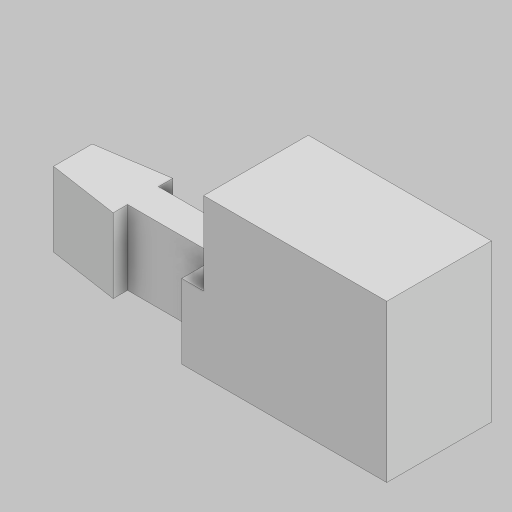
# Autodesk Inventor part: Tenon2
Saved by Autodesk Inventor 2023 (Build 270158000, 158)
## iProperties
Created: 2026-02-15
Part Number: Tenon2
Material: Genérico
Document SubType Name: Modeling
Designer: MARTIN MAESTRE
Density: 1 g/cm^3
Appearance: Valor por defecto
Author: MARTIN MAESTRE
Autodesk Inventor part; units mm, degrees
ref_plane "YZ Plane" through (0, 0, 0) normal (1, 0, 0) x (0, 1, 0)
ref_plane "XZ Plane" through (0, 0, 0) normal (0, 1, 0) x (-1, 0, 0)
ref_plane "XY Plane" through (0, 0, 0) normal (0, 0, 1) x (1, 0, 0)
sketch "Boceto1" plane through (0, 0, 0) normal (0, 0, 1) x (1, 0, 0)
  line L0 (0, 0) -> (140, 0)
  line L1 (140, 0) -> (140, 60)
  line L2 (140, 60) -> (0, 60)
  line L3 (0, 60) -> (0, 0)
  dimension "d0" = 140
  dimension "d1" = 60
  constraints: 8 end point, 3 perpendicular, 1 horizontal
  measures "d0" distance of L0.start L0.end
  measures "d1" distance of L0.end L1.end
extrude "Extrusión1" add sketch "Boceto1" along normal blind 40
sketch "Boceto2" plane through (0, 60, 0) normal (0, 1, 0) x (1, 0, 0)
  line L0 (140, -40) -> (0, -40) projected
  line L1 (0, 0) -> (0, -40)
  line L2 (140, 0) -> (0, 0) projected
  line L3 (0, 0) -> (70, 0)
  line L4 (0, 0) -> (70, 0) construction
  line L5 (70, 0) -> (70, -40)
  line L6 (0, -40) -> (70, -40)
  dimension "d4" = 70
  dimension "d5" = 0
  constraints: 10 end point, 3 collinear, 1 horizontal, 1 midpoint, 1 vertical
  measures "d4" distance of L1.start L3.end
  measures "d5" distance between parallel lines of L3 L4
extrude "Extrusión2" cut sketch "Boceto2" against normal blind 31.6
sketch "Boceto3" plane through (0, 0, 0) normal (0, -1, 0) x (1, 0, 0)
  line L0 (0, 0) -> (140, 0) projected
  line L1 (0, 0) -> (0, 12.6)
  line L2 (0, 0) -> (0, 40) projected
  line L3 (0, 12.6) -> (0, 27.4) construction
  line L4 (0, 27.4) -> (0, 40)
  line L5 (0, 0) -> (26.8, 0)
  line L6 (26.8, 0) -> (26.8, 8.6) construction
  line L7 (0, 12.6) -> (26.8, 8.6)
  line L8 (26.8, 0) -> (26.8, 8.6)
  line L9 (26.8, 8.6) -> (26.8, 14.1)
  line L10 (26.8, 14.1) -> (61.6, 14.1)
  line L11 (26.8, 0) -> (61.6, 0)
  line L12 (61.6, 0) -> (61.6, 14.1)
  line L13 (0, 40) -> (140, 40) projected
  line L14 (0, 40) -> (61.6, 40)
  line L15 (61.6, 40) -> (61.6, 25.9)
  line L16 (61.6, 25.9) -> (26.8, 25.9)
  line L17 (61.6, 25.9) -> (96.4, 25.9) construction
  line L18 (26.8, 25.9) -> (26.8, 31.4)
  line L19 (26.8, 31.4) -> (0, 27.4)
  dimension "d8" = 12.6
  dimension "d9" = 14.8
  dimension "d10" = 26.8
  dimension "d11" = 8.6
  dimension "d12" = 5.5
  dimension "d13" = 34.8
  dimension "d14" = 14.1
  dimension "d15" = 61.6
  dimension "d16" = 34.8
  dimension "d17" = 180
  dimension "d18" = 5.5
  constraints: 34 end point, 5 point on line, 4 perpendicular, 3 vertical, 2 collinear, 2 horizontal
  measures "d8" distance of L0.start L1.end
  measures "d9" distance of L1.end L3.end
  measures "d10" distance of L0.start L5.end
  measures "d11" distance of L5.end L6.end
  measures "d12" distance of L6.end L9.end
  measures "d13" distance of L9.end L10.end
  measures "d14" distance of L14.end L15.end
  measures "d15" distance between parallel lines of L2 L15
  measures "d16" distance of L15.end L16.end
  measures "d17" angle of L16 L17
  measures "d18" distance of L16.end L18.end
extrude "Extrusión3" cut sketch "Boceto3" against normal blind 30
